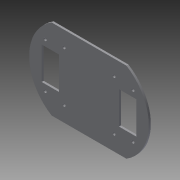
# Autodesk Inventor part: base
Saved by Autodesk Inventor 2014 SP1 (Build 180222100, 222)
## iProperties
Created: 2014-09-21
Part Number: base
Material: Générique
Document SubType Name: Modeling
Designer: astralien3000
Density: 1 g/cm^3
Appearance: Par défaut
Author: astralien3000
Autodesk Inventor part; units mm, degrees
ref_plane "YZ Plane" through (0, 0, 0) normal (1, 0, 0) x (0, 1, 0)
ref_plane "XZ Plane" through (0, 0, 0) normal (0, 1, 0) x (-1, 0, 0)
ref_plane "XY Plane" through (0, 0, 0) normal (0, 0, 1) x (1, 0, 0)
sketch "Esquisse1" plane through (0, 0, 0) normal (0, 1, 0) x (-1, 0, 0)
  circle A0 centre (0, 0) radius 25 construction
  line L0 (-25, 0) -> (25, 0) construction
  arc A1 (-75, -80.7775) -> (-75, 80.7775) centre (-25, 0) ccw construction
  arc A2 (75, 80.7775) -> (75, -80.7775) centre (25, 0) ccw construction
  line L1 (0, 25) -> (0, 0) construction
  line L2 (-75, 80.7775) -> (75, 80.7775)
  line L3 (-75, -80.7775) -> (75, -80.7775)
  arc A3 (75, -80.7775) -> (75, 80.7775) centre (25, 0) ccw
  arc A4 (-75, 80.7775) -> (-75, -80.7775) centre (-25, 0) ccw
  dimension "d0" = 50
  dimension "d1" = 190
  dimension "d2" = 150
  constraints: 11 point on circle, 8 end point, 5 centre point, 3 coincident, 2 perpendicular, 1 horizontal, 1 midpoint, 2 other
  measures "d0" diameter of A0
  measures "d1" diameter of A1
  measures "d2" distance of L2.start L2.end
extrude "Extrusion1" add sketch "Esquisse1" along normal blind 4
sketch "Esquisse2" plane through (0, 4, 0) normal (0, 1, 0) x (1, 0, 0)
  line L0 (75, 80.7775) -> (-75, 80.7775) projected
  arc A0 (-75, 80.7775) -> (-75, -80.7775) centre (-25, 0) ccw projected
  line L1 (-95, 32.5) -> (-60, 32.5)
  line L2 (-60, 32.5) -> (-60, -32.5)
  line L3 (-60, -32.5) -> (-95, -32.5)
  line L4 (-95, -32.5) -> (-95, 32.5)
  line L5 (60, 32.5) -> (95, 32.5)
  line L6 (95, 32.5) -> (95, -32.5)
  line L7 (95, -32.5) -> (60, -32.5)
  line L8 (60, -32.5) -> (60, 32.5)
  line L9 (0, 0) -> (0, 80.7775) construction
  line L10 (0, 0) -> (-120, 0) construction
  dimension "d5" = 35
  dimension "d6" = 60
  dimension "d7" = 65
  constraints: 20 end point, 4 parallel, 2 horizontal, 2 perpendicular, 1 midpoint, 1 point on circle, 5 other
  measures "d5" distance between parallel lines of L4 L2
  measures "d6" distance between parallel lines of L9 L2
  measures "d7" distance between parallel lines of L1 L3
extrude "Extrusion2" cut sketch "Esquisse2" against normal through all
sketch "Esquisse3" plane through (0, 4, 0) normal (0, 1, 0) x (1, 0, 0)
  line L0 (75, 80.7775) -> (-75, 80.7775) projected
  circle A0 centre (-88, 45) radius 3
  circle A1 centre (-88, -45) radius 3
  line L1 (-88, -45) -> (-88, 45) construction
  line L2 (0, 0) -> (-88, 0) construction
  line L3 (0, 0) -> (0, 80.7775) construction
  circle A2 centre (88, 45) radius 3
  circle A3 centre (88, -45) radius 3
  dimension "d10" = 88
  dimension "d11" = 6
  dimension "d12" = 90
  constraints: 6 end point, 4 centre point, 2 midpoint, 2 perpendicular, 2 symmetric about line, 3 other
  measures "d10" distance between parallel lines of L3 L1
  measures "d11" diameter of A0
  measures "d12" distance of L1.start L1.end
extrude "Extrusion3" cut sketch "Esquisse3" against normal through all
sketch "Esquisse4" plane through (0, 0, 0) normal (0, -1, 0) x (1, 0, 0)
  line L0 (-50, 50) -> (50, 50) construction
  line L1 (50, 50) -> (50, -50) construction
  line L2 (50, -50) -> (-50, -50) construction
  line L3 (-50, -50) -> (-50, 50) construction
  circle A0 centre (-50, 50) radius 3
  circle A1 centre (50, 50) radius 3
  circle A2 centre (50, -50) radius 3
  circle A3 centre (-50, -50) radius 3
  line L4 (75, 80.7775) -> (-75, 80.7775) projected
  point P0 (0, 0)
  dimension "d15" = 100
  dimension "d16" = 100
  dimension "d17" = 50
  dimension "d18" = 50
  dimension "d19" = 6
  dimension "d20" = 6
  dimension "d21" = 6
  dimension "d22" = 6
  dimension "d25" = 30.7775
  constraints: 8 end point, 4 centre point, 4 coincident, 2 parallel, 1 horizontal, 1 perpendicular
  measures "d15" distance of L0.end L1.end
  measures "d16" distance of L0.start L0.end
  measures "d17" distance from line of L1 point (0, 0)
  measures "d18" distance from line of L2 point (0, 0)
  measures "d19" diameter of A0
  measures "d20" diameter of A1
  measures "d21" diameter of A2
  measures "d22" diameter of A3
  measures "d25" distance between parallel lines of L4 L0
extrude "Extrusion4" cut sketch "Esquisse4" against normal through all
equation "\"d17\" = 0.5 * d16"
equation "\"d18\" = 0.5 * d15"
equation "\"d20\" = d19"
equation "\"d21\" = d19"
equation "\"d22\" = d19"
